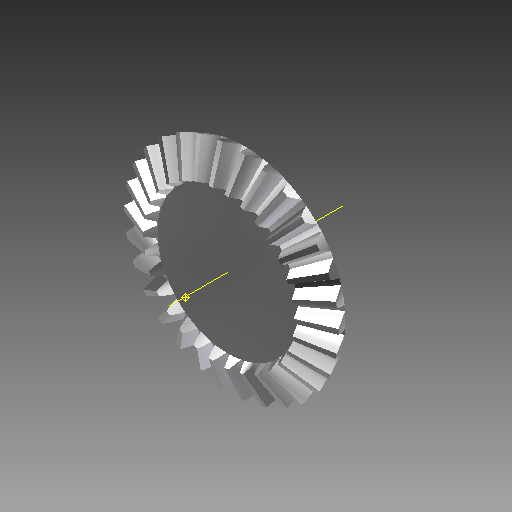
# Autodesk Inventor part: Bevel Gear1
Saved by Autodesk Inventor 2019.4 (Build 234330000, 330)
## iProperties
Created: 2019-11-29
Part Number: Bevel Gear1
Material: Aluminum 6061
Document SubType Name: Modeling
Designer: admin
Categories: <?xml version="1.0" encoding="UTF-16"?> <MemberInstance><Categories><FamilyTemplate><FamilyTemplateParameter ValueType="xs:double" Id="1" ObjectReferenceKey="da_z" ObjectType="kUserParameterObject"/><FamilyTemplateParameter ValueType="xs:double" Id="2" ObjectReferenceKey="da_b" ObjectType="kUserParameterObject"/><FamilyTemplateParameter ValueType="xs:double" Id="3" ObjectReferenceKey="da_beta" ObjectType="kUserParameterObject"/><FamilyTemplateParameter ValueType="xs:double" Id="4" ObjectReferenceKey="da_dae" ObjectType="kUserParameterObject"/><FamilyTemplateParameter ValueType="xs:double" Id="5" ObjectReferenceKey="da_ve" ObjectType="kUserParameterObject"/><FamilyTemplateParameter ValueType="xs:double" Id="6" ObjectReferenceKey="da_omega" ObjectType="kUserParameterObject"/><FamilyTemplateParameter ValueType="xs:string" Id="7" ObjectReferenceKey="EAIAABAAAAAAHwAAAAAAAIAAAAAAAAAA" ObjectType="83914240" SubObjectId="SurfaceGeometry"/></FamilyTemplate><ParamToTemplateMap><ParamToTemplate CategoryParameter="//CategoryParameter[@InternalName='046C89C9-8512-4d59-83FE-43B91F4F132A']" TemplateParameter="1"/><ParamToTemplate CategoryParameter="//CategoryParameter[@InternalName='2552DF32-E462-4b46-AEBF-C6C7768E72AC']" TemplateParameter="2"/><ParamToTemplate CategoryParameter="//CategoryParameter[@InternalName='C9EE641D-15FC-4fae-A226-E94C4372FDD7']" TemplateParameter="3"/><ParamToTemplate><ParamToTemplate CategoryParameter="//CategoryParameter[@InternalName='00B6519A-459B-49c7-AD84-2E56D39A5744']" ConstantValue="0.300000"/></ParamToTemplate><ParamToTemplate><ParamToTemplate CategoryParameter="//CategoryParameter[@InternalName='04B31F0E-C7A6-4894-AA32-9629BEFACF47']" ConstantValue="1.000000"/></ParamToTemplate><ParamToTemplate><ParamToTemplate CategoryParameter="//CategoryParameter[@InternalName='43CBEC2E-7847-49e7-A936-2F7889FCB2D9']" ConstantValue="0.200000"/></ParamToTemplate><ParamToTemplate><ParamToTemplate CategoryParameter="//CategoryParameter[@InternalName='B1EFC894-105D-4ebd-86BF-FA20ED196853']" ConstantValue="0.300000"/></ParamToTemplate><ParamToTemplate><ParamToTemplate CategoryParameter="//CategoryParameter[@InternalName='51175063-3D10-4879-93E8-6246FE8B403D']" ConstantValue="2060000000.000000"/></ParamToTemplate><ParamToTemplate><ParamToTemplate CategoryParameter="//CategoryParameter[@InternalName='A3A52E27-4454-46a9-B0BD-C932399B70AF']" ConstantValue="0.300000"/></ParamToTemplate><ParamToTemplate CategoryParameter="//CategoryParameter[@InternalName='2A200944-5A8C-41ca-B96E-8520D2E510F1']" TemplateParameter="4"/><ParamToTemplate><ParamToTemplate CategoryParameter="//CategoryParameter[@InternalName='1A637F62-92C8-44bc-B81F-10802510B579']" ConstantValue="4.374363"/></ParamToTemplate><ParamToTemplate CategoryParameter="//CategoryParameter[@InternalName='B52DD4BE-6863-48fb-BF58-89EF6F9EC65C']" TemplateParameter="5"/><ParamToTemplate><ParamToTemplate CategoryParameter="//CategoryParameter[@InternalName='3956BFF2-84D2-457d-93C2-9B0613DEBA67']" ConstantValue="0.889569"/></ParamToTemplate><ParamToTemplate CategoryParameter="//CategoryParameter[@InternalName='739CFA02-461B-4bf8-8049-181FCAD8B28F']" TemplateParameter="6"/><ParamToTemplate><ParamToTemplate CategoryParameter="//CategoryParameter[@InternalName='A27E999F-E2CE-4481-8A2A-EBF499C4C3C5']" ConstantValue="0.000000"/></ParamToTemplate><ParamToTemplate><ParamToTemplate CategoryParameter="//CategoryParameter[@InternalName='9E1B4470-B2D3-4ff1-B813-535BB4CDF51A']" ConstantValue="3520000.000000"/></ParamToTemplate><ParamToTemplate><ParamToTemplate CategoryParameter="//CategoryParameter[@InternalName='F8452263-BFF6-458c-9FB1-07C4B99E95CD']" ConstantValue="11400000.000000"/></ParamToTemplate><ParamToTemplate><ParamToTemplate CategoryParameter="//CategoryParameter[@InternalName='3E3BB259-FD49-497f-8171-6EBC954A3479']" ConstantValue="2.000000"/></ParamToTemplate><ParamToTemplate CategoryParameter="//CategoryParameter[@InternalName='27C3BAF2-7550-4e4b-AE2C-0DB134B7D9B7']" TemplateParameter="7"/></ParamToTemplateMap><Category DisplayName="Gear" InternalName="DC85795E-93AB-48d5-8EEE-5A27447B64BD" Mnemonic="Gear"><CategoryParameter DisplayName="z" InternalName="046C89C9-8512-4d59-83FE-43B91F4F132A" Mnemonic="z"/><CategoryParameter DisplayName="b" InternalName="2552DF32-E462-4b46-AEBF-C6C7768E72AC" Mnemonic="b"/><CategoryParameter DisplayName="||b|" InternalName="C9EE641D-15FC-4fae-A226-E94C4372FDD7" Mnemonic="beta"/><CategoryParameter DisplayName="x" InternalName="00B6519A-459B-49c7-AD84-2E56D39A5744" Mnemonic="x"/><CategoryParameter DisplayName="a*" InternalName="04B31F0E-C7A6-4894-AA32-9629BEFACF47" Mnemonic="a"/><CategoryParameter DisplayName="c*" InternalName="43CBEC2E-7847-49e7-A936-2F7889FCB2D9" Mnemonic="c"/><CategoryParameter DisplayName="r|.f|*" InternalName="B1EFC894-105D-4ebd-86BF-FA20ED196853" Mnemonic="rf"/><CategoryParameter DisplayName="E" InternalName="51175063-3D10-4879-93E8-6246FE8B403D" Mnemonic="E"/><CategoryParameter DisplayName="||m|" InternalName="A3A52E27-4454-46a9-B0BD-C932399B70AF" Mnemonic="mi"/><Category DisplayName="BevelGear" InternalName="0C98F69A-0C2B-4791-B2FE-7691BB227E77" Mnemonic="BevelGear"><CategoryParameter DisplayName="d|.ae|" InternalName="2A200944-5A8C-41ca-B96E-8520D2E510F1" Mnemonic="dae"/><CategoryParameter DisplayName="d|.ai|" InternalName="1A637F62-92C8-44bc-B81F-10802510B579" Mnemonic="dai"/><CategoryParameter DisplayName="A|.e|" InternalName="B52DD4BE-6863-48fb-BF58-89EF6F9EC65C" Mnemonic="ve"/><CategoryParameter DisplayName="A|.i|" InternalName="3956BFF2-84D2-457d-93C2-9B0613DEBA67" Mnemonic="vi"/><CategoryParameter DisplayName="||S|" InternalName="739CFA02-461B-4bf8-8049-181FCAD8B28F" Mnemonic="omega"/><CategoryParameter DisplayName="x|.t|" InternalName="A27E999F-E2CE-4481-8A2A-EBF499C4C3C5" Mnemonic="xt"/><CategoryParameter DisplayName="||s||.Flim|" InternalName="9E1B4470-B2D3-4ff1-B813-535BB4CDF51A" Mnemonic="sFlim"/><CategoryParameter DisplayName="||s||.Hlim|" InternalName="F8452263-BFF6-458c-9FB1-07C4B99E95CD" Mnemonic="sHlim"/><CategoryParameter DisplayName="type" InternalName="3E3BB259-FD49-497f-8171-6EBC954A3479" Mnemonic="type"/><CategoryParameter DisplayName="PitchDiameter" InternalName="27C3BAF2-7550-4e4b-AE2C-0DB134B7D9B7" Mnemonic="IDS_PITCHDIAM"/></Category></Category></Categories></MemberInstance>
Mass: 34.6047 g
Surface Area: 78.1273 cm^2
Volume: 12.8165 cm^3
Density: 2.7 g/cm^3
Appearance: Aluminum - Flat
CustomPartVersion: 1
Author: admin
Autodesk Inventor part; units mm, degrees
ref_plane "Mesh Plane2" through (0, 0, 0) normal (0.9945219, 0.1045285, 0) x (0, 0, 1)
sketch "Teeth Body Sketch" plane through (0, 0, 0) normal (1, 0, 0) x (0, 1, 0)
  line L0 (0, 0) -> (29.195016, -16.609969) construction
  line L1 (29.195016, -16.609969) -> (31.162755, -12.674489)
  line L2 (31.162755, -12.674489) -> (0, 0) construction
  line L3 (30, -15) -> (0, 0) construction
  line L4 (20.490744, -11.657833) -> (21.871817, -8.895687)
  line L5 (29.195016, -16.609969) -> (20.490744, -11.657833)
  line L6 (31.162755, -12.674489) -> (21.871817, -8.895687)
  line L7 (0, -14.948972) -> (0, 2.491495)
  line L8 (0, -15) -> (31.162755, -15) construction
  dimension "d0" = 60
  dimension "d1" = 58.39003
  dimension "d2" = 62.32551
  dimension "d3" = 10
  dimension "d4" = 12.67449
  constraints: 16 end point, 4 point on line, 3 perpendicular, 2 collinear, 1 horizontal alignment, 1 vertical alignment
  measures "d0" diameter of L3.start L7
  measures "d1" diameter of L0.end L7
  measures "d2" diameter of L1.end L7
  measures "d3" distance between parallel lines of L1 L4
  measures "d4" vertical distance of L1.end L0.start
revolve "Teeth Body" add sketch "Teeth Body Sketch" angle 360 about axis through (0, 0, 0) along (0, 0, 1)
ref_plane "Tooth Plane" through (0, 30, -15) normal (0, -0.8944272, 0.4472136) x (1, 0, 0)
sketch "Start Sketch" plane through (0, 30, -15) normal (0, -0.8944272, 0.4472136) x (1, 0, 0)
  line L0 (0, -60.963874) -> (0, 13.602536)
  arc A0 (-0.615438, -2.327999) -> (-3.220099, 3.846944) centre (-25.018181, -8.984542) ccw
  arc A1 (3.220099, 3.846944) -> (0.615438, -2.327999) centre (25.018181, -8.984542) ccw
  line L1 (-0.615438, -2.327999) -> (0.615438, -2.327999)
  arc A2 (3.220099, 3.846944) -> (-3.220099, 3.846944) centre (0, -67.082039) ccw
  dimension "d7" = 25.29434
  dimension "d8" = 25.01818
  dimension "d9" = 58.0975
  dimension "d57" = 71.00204
  dimension "d58" = 64.75404
  constraints: 6 point on circle, 3 centre point, 3 symmetric about line, 2 end point, 1 coincident, 1 perpendicular, 1 other
  measures "d7" radius of A0
  measures "d8" horizontal distance of point (0, -67.082) A0.centre
  measures "d9" vertical distance of point (0, -67.082) A0.centre
  measures "d57" radius of A2
  measures "d58" distance from line of A2.centre L1
sketch "End Sketch" plane through (0, 20.858954, -10.429477) normal (0, -0.8944272, 0.4472136) x (1, 0, 0)
  line L0 (0, -36.340102) -> (0, 8.169906)
  arc A0 (-0.428529, -1.553901) -> (-2.24215, 2.745703) centre (-17.420121, -6.188841) ccw
  arc A1 (2.24215, 2.745703) -> (0.428529, -1.553901) centre (17.420121, -6.188841) ccw
  line L1 (-0.428529, -1.553901) -> (0.428529, -1.553901)
  arc A2 (2.24215, 2.745703) -> (-2.24215, 2.745703) centre (0, -46.642039) ccw
  dimension "d12" = 17.61241
  dimension "d15" = 17.42012
  dimension "d16" = 40.4532
  dimension "d59" = 49.43861
  dimension "d60" = 45.08814
  constraints: 6 point on circle, 3 centre point, 3 symmetric about line, 2 end point, 1 coincident, 1 other
  measures "d12" radius of A0
  measures "d15" horizontal distance of A0.centre point (0, -46.642)
  measures "d16" vertical distance of A0.centre point (0, -46.642)
  measures "d59" radius of A2
  measures "d60" distance from line of A2.centre L1
loft "Loft" cut profiles "Start Sketch", "End Sketch"
pattern_circular "Circular Pattern" count 30 over 360 about axis through (0, 0, 0) along (0, 0, 1) of "Loft"
ref_plane "End Plane" through (0, 20.858954, -10.429477) normal (0, -0.8944272, 0.4472136) x (1, 0, 0)
sketch3d "3D Sketch Right"
ref_plane "End Plane Right" through (-1.773617, 20.783413, -10.429477) normal (0.0760523, -0.891188, 0.4472136) x (0.9963785, 0.0850291, 0)
sketch "End Sketch Right" plane through (-1.773617, 20.783413, -10.429477) normal (0.0760523, -0.891188, 0.4472136) x (0.9963785, 0.0850291, 0)
  arc A0 (-0.428529, -1.553901) -> (-2.24215, 2.745703) centre (-17.420121, -6.188841) ccw
  line L0 (0, -57.520932) -> (0, 12.690226)
  arc A1 (2.24215, 2.745703) -> (0.428529, -1.553901) centre (17.420121, -6.188841) ccw
  line L1 (-0.428529, -1.553901) -> (0.428529, -1.553901)
  arc A2 (2.24215, 2.745703) -> (-2.24215, 2.745703) centre (0, -46.642039) ccw
  dimension "d70" = 17.42012
  dimension "d71" = 40.4532
  dimension "d72" = 17.61241
  dimension "d73" = 45.08814
  dimension "d74" = 49.43861
  constraints: 6 point on circle, 3 centre point, 3 symmetric about line, 2 end point, 1 coincident, 1 perpendicular, 1 other
  measures "d70" horizontal distance of A2.centre A0.centre
  measures "d71" vertical distance of point (0, -46.642) A0.centre
  measures "d72" radius of A0
  measures "d73" distance from line of point (0, -46.642) L1
  measures "d74" radius of A2
feature "Loft Right" [suppressed]
pattern_circular "Circular Pattern Right" [suppressed]
sketch3d "3D Sketch Left"
ref_plane "End Plane Left" through (1.843957, 20.783413, -10.457399) normal (-0.0790076, -0.8905025, 0.448066) x (0.9960872, -0.0883754, 0)
sketch "End Sketch Left" plane through (1.843957, 20.783413, -10.457399) normal (-0.0790076, -0.8905025, 0.448066) x (0.9960872, -0.0883754, 0)
  line L0 (0, -57.8638) -> (0, 13.068646)
  arc A0 (-0.428529, -1.53165) -> (-2.24215, 2.767954) centre (-17.420121, -6.16659) ccw
  arc A1 (2.24215, 2.767954) -> (0.428529, -1.53165) centre (17.420121, -6.16659) ccw
  line L1 (-0.428529, -1.53165) -> (0.428529, -1.53165)
  ellipse E0 centre (0, -7.952748) end of major axis (21.871817, -7.952748) minor radius 9.800017
  arc A2 (2.24215, 2.767954) -> (-2.24215, 2.767954) centre (0, -46.619788) ccw
  dimension "d56" = 9.80002
  dimension "d30" = 17.61241
  dimension "d31" = 17.42012
  dimension "d32" = 40.4532
  dimension "d61" = 49.43861
  dimension "d62" = 45.08814
  constraints: 6 point on circle, 3 centre point, 3 symmetric about line, 2 end point, 1 coincident, 2 other
  measures "d30" radius of A0
  measures "d31" horizontal distance of point (0, -46.62) A0.centre
  measures "d32" vertical distance of A0.centre point (0, -46.62)
  measures "d61" radius of A2
  measures "d62" distance from line of point (0, -46.62) L1
feature "Loft Left" [suppressed]
pattern_circular "Circular Pattern Left" [suppressed]
sketch "Body Sketch" plane through (0, 0, 0) normal (1, 0, 0) x (0, 1, 0)
  line L0 (0, -13.447904) -> (0, -6.514914)
  line L1 (29.195016, -16.609969) -> (20.490744, -11.657833)
  line L2 (20.490744, -11.657833) -> (0, -11.657833)
  line L3 (29.195016, -16.609969) -> (0, -16.609969)
  constraints: 4 end point, 2 perpendicular, 2 point on line
sketch "Body Sketch outline for Fix Body" plane through (0, 0, 0) normal (1, 0, 0) x (0, 1, 0)
  line L0 (0, -16.609969) -> (29.195016, -16.609969)
  line L1 (0, -11.657833) -> (0, -16.609969)
  line L2 (20.490744, -11.657833) -> (0, -11.657833)
  line L3 (29.195016, -16.609969) -> (20.490744, -11.657833)
revolve "Fix Body" add sketch "Body Sketch outline for Fix Body" angle 360 about axis through (0, 0, 0) along (0, 0, 1)
sketch "Sketch6" plane through (0, 0, 0) normal (1, 0, 0) x (0, 1, 0)
  line L0 (30, -15) -> (0, 0) projected
  line L1 (0, -13.5) -> (0, 2.25) projected
surface revolve "Pitch Diameter" sketch "Sketch6" angle 360 about axis through (0, 0, 0) along (0, 0, 1) shown no curves L0
equation "\"d0\" = da_de"
equation "\"d1\" = da_dfe"
equation "\"d2\" = da_dae"
equation "\"d3\" = da_b"
equation "\"d4\" = da_ve"
equation "\"d7\" = fd_rr"
equation "\"d8\" = fd_x"
equation "\"d9\" = fd_y"
equation "\"d57\" = 0.5 * fd_dva + 0.3 * da_he"
equation "\"d58\" = 0.5 * fd_dva - 1.12 * da_he"
equation "\"da_teethtype\" = 0"
equation "\"da_b\" = 10"
equation "\"da_de\" = 60"
equation "\"da_dae\" = 62.32551"
equation "\"da_dfe\" = 58.39003"
equation "\"da_le\" = 33.54102"
equation "\"da_omega\" = 90deg"
equation "\"da_beta\" = 0"
equation "\"da_delta\" = 63.434949deg"
equation "\"da_alpha\" = 20deg"
equation "\"da_he\" = 4.4"
equation "\"da_ve\" = 12.67449"
equation "\"da_zv\" = 67.082039"
equation "\"fd_loft\" = da_b + 0.05 * da_he"
equation "\"fd_x\" = fd_x1 + fd_x2"
equation "\"fd_y\" = fd_y1 - fd_y2"
equation "\"fd_dd\" = fd_dva - 0.8 * da_he"
equation "\"da_dvw\" = 135.36408"
equation "\"d11\" = fd_loft"
equation "\"da_dm\" = 51.05573"
equation "\"da_x\" = 0.3"
equation "\"da_m\" = 2"
equation "\"d50\" = da_omega"
equation "\"fd_rr\" = 25.294336"
equation "\"fd_dva\" = 139.364079"
equation "\"fd_x1\" = 1.602306"
equation "\"fd_x2\" = 23.415876"
equation "\"fd_y1\" = 67.66307"
equation "\"fd_y2\" = 9.565573"
body "Solid1"
body "Srf1"
